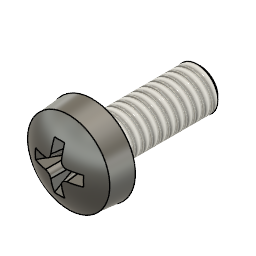
Empty (Autodesk Fusion 360 archive; units mm, degrees)
design "Raised Cheese Head Screw DIN 7985 - M2 x 5 - H Steel 4.6 Plain"
description: Raised Cheese Head Screw DIN 7985 - M2 x 5 - H
part number: DIN 7985 - M2x5-H H Steel 4.6 Plain
Autodesk Fusion 360 part; units mm, degrees
sketch "Sketch1" plane through (0, 0, 0) normal (0, 1, 0) x (1, 0, 0)
  line L0 (-1, 5) -> (0, 5)
  line L1 (0, 5) -> (0, -1.72)
  line L2 (-0.9, 0) -> (-2, 0)
  line L3 (-2, 0) -> (-1.9045, -1.0916)
  arc A0 (-1.9045, -1.0916) -> (0, -1.72) centre (0, 1.48) ccw
  line L4 (-0.9, 0) -> (-0.9, 0.64)
  line L5 (-0.9, 0.64) -> (-1, 0.64)
  line L6 (-1, 0.64) -> (-1, 5)
  dimension "d66" = 4
  dimension "d79" = 2
  dimension "d81" = 1.8
  dimension "d84" = 0.64
  dimension "d85" = 85
  dimension "d107" = 1.72
  dimension "d108" = 5
  dimension "d109" = 3.52
  constraint collinear origin L1.end L0.end
  constraint coincident origin L2
  constraint vertical L1
  constraint coincident L1 A0.centre
  constraint perpendicular L2 L4
  constraint perpendicular L4 L5
  constraint perpendicular L0 L6
  constraint coincident L0.start L6.end
  constraint vertical L6
  constraint vertical L4
  measures "d84" distance of L2 L5
  measures "d85" angle of L2 L3
  measures "d107" distance of L1.end L2
  measures "d108" distance of origin L0
  measures "d109" distance of L0 A0.centre
revolve "Revolve1" add sketch "Sketch1" angle 360 about axis through (0, 0, -5) along (0, 0, 1) makes body 1
ref_plane "WorkPlane1" through (0, 0, 1.72) normal (0, 0, 1) x (1, 0, 0)
sketch "Sketch2" plane through (0, 0, 1.72) normal (0, 0, 1) x (1, 0, 0)
  line L0 (-0.25, 0.25) -> (-1.25, 0.25)
  line L1 (-0.25, -0.25) -> (-1.25, -0.25)
  line L2 (-1.25, 0.25) -> (-1.25, -0.25)
  line L3 (-0.25, -0.25) -> (-0.25, -1.25)
  line L4 (-0.25, -1.25) -> (0.25, -1.25)
  line L5 (0.25, -0.25) -> (0.25, -1.25)
  line L6 (0.25, -0.25) -> (1.25, -0.25)
  line L7 (1.25, -0.25) -> (1.25, 0.25)
  line L8 (0.25, 0.25) -> (1.25, 0.25)
  line L9 (0.25, 0.25) -> (0.25, 1.25)
  line L10 (0.25, 1.25) -> (-0.25, 1.25)
  line L11 (-0.25, 0.25) -> (-0.25, 1.25)
  dimension "d101" = 0.5
  dimension "d103" = 360
  dimension "d104" = 2.5
  constraint vertical L0.start L1.start
  constraint vertical L2
  constraint horizontal L0
  constraint coincident L0.start L11.start
  measures "d101" distance of L0 L1
  measures "d104" distance of L2 L7
extrude "Extrude1" add sketch "Sketch2" against normal blind 1 draft -4 separate body makes body 2
draft "Draft1" angle -30 neutral plane through (0, 0, 1.72) pull (0, 0, 1) 4 faces at (-1.2267, -0.06, 1.3867) (0.06, -1.2267, 1.3867) (1.2267, 0.06, 1.3867) (-0.06, 1.2267, 1.3867) on bodies 2
fillet "Fillet3" radius 0.25 4 edges at (-0.215, -0.215, 1.22) (0.215, -0.215, 1.22) (-0.215, 0.215, 1.22) (0.215, 0.215, 1.22) on bodies 2
combine "Combine1" operation cut target body 1 tool bodies 2
thread "Thread2" "ISO Metric profile 2.0 M2x0.4 M2x0.4 6g" major diameter 1.9335 minor diameter 1.478 pitch 0.4 angle 60 resizes the face on face at (-0.9988, 0.0498, -3.5467) on bodies 1
sketch "Sketch5" plane through (0, 0, 0) normal (0, 1, 0) x (1, 0, 0)
  line L0 (0, 5) -> (0, -1.72)
  line L1 (0, 5) -> (-1.02, 5)
  line L2 (-1.02, 5) -> (-1.02, 4.8)
  line L3 (-1.02, 4.8) -> (-0.82, 5)
  dimension "d93" = 45
  dimension "d110" = 1.02
  dimension "d111" = 0.2
  constraint coincident L0.start L1.start
  constraint perpendicular L0 L1
  constraint perpendicular L1 L2
  constraint coincident L1 L3.end
  measures "d93" angle of L2 L3
  measures "d110" distance of L0.start L2
  measures "d111" distance of L2 L3.end
revolve "Revolve2" cut sketch "Sketch5" angle 360 about axis through (0, 0, 1.75) along (0, 0, 1) bodies 1
equation "adsk_nomlen = 5.00 mm"
equation "adsk_headh = 1.72 mm"
equation "adsk_headdia = 4.00 mm"
equation "adsk_nomdia = 2.00 mm"
equation "adsk_phildia = 2.50 mm"
equation "d31 = -adsk_phildepth"
equation "adsk_phildepth = 1.00 mm"
equation "d66 = adsk_headdia"
equation "d71 = adsk_headh"
equation "adsk_thrlen = 4.36 mm"
equation "d79 = adsk_nomdia"
equation "d81 = adsk_nomdia - ( adsk_pitch1 / 2 )"
equation "adsk_pitch1 = 0.40 mm"
equation "d84 = adsk_nomlen - adsk_thrlen"
equation "adsk_philwidth = adsk_phildia / 5"
equation "d101 = adsk_philwidth"
equation "d104 = adsk_phildia"
equation "d106 = adsk_phildia * 0.1"
equation "d107 = adsk_headh"
equation "d108 = adsk_nomlen"
equation "d109 = ( adsk_nomlen + adsk_headh ) - ( adsk_headdia * 0.8 )"
equation "d110 = adsk_nomdia * 0.51"
equation "d111 = adsk_pitch1 / 2"
